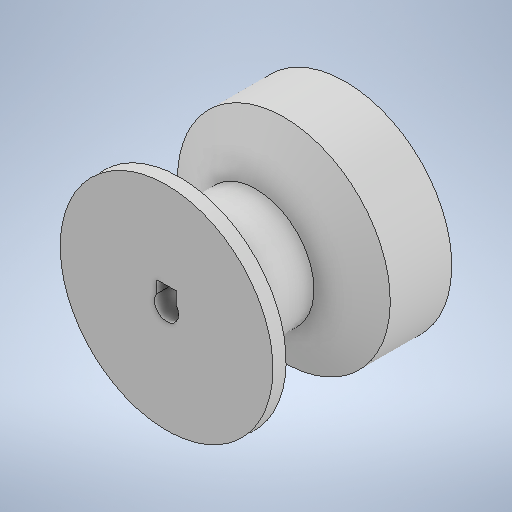
# Autodesk Inventor part: Vbelt Drive Pulley
Saved by Autodesk Inventor 2025 (Build 290162010, 162A)
## iProperties
Created: 2024-08-22
Part Number: Vbelt Drive Pulley
Material: Generic
Document SubType Name: Modeling
Designer: max_d
Density: 1 g/cm^3
Appearance: Default
Author: max_d
Autodesk Inventor part; units mm, degrees
ref_plane "YZ Plane" through (0, 0, 0) normal (1, 0, 0) x (0, 1, 0)
ref_plane "XZ Plane" through (0, 0, 0) normal (0, 1, 0) x (-1, 0, 0)
ref_plane "XY Plane" through (0, 0, 0) normal (0, 0, 1) x (1, 0, 0)
sketch "Sketch2" plane through (0, 0, 0) normal (1, 0, 0) x (0, 1, 0)
  line L0 (0, 0) -> (12, 0) construction
  line L1 (12, 0) -> (12, -5)
  line L2 (12, -5) -> (22, -10.7735)
  line L3 (22, -10.7735) -> (22, -13.5)
  line L4 (22, -13.5) -> (0, -13.5)
  line L5 (0, -13.5) -> (0, 0)
  line L6 (12, 0) -> (12, 5)
  line L7 (12, 5) -> (22, 10.7735)
  line L8 (22, 10.7735) -> (22, 13.5)
  line L9 (22, 13.5) -> (0, 13.5)
  line L10 (0, 13.5) -> (0, 0)
  line L11 (0, 0) -> (0, -46.5785) construction
  line L12 (22, -13.5) -> (22, -23.5)
  line L13 (22, -23.5) -> (0, -23.5)
  line L14 (0, -13.5) -> (0, -23.5)
  dimension "d0" = 22
  dimension "d1" = 13.5
  dimension "d2" = 5
  dimension "d3" = 60
  dimension "d4" = 10
  dimension "d16" = 10
  constraints: 30 end point, 4 symmetric about line, 3 perpendicular, 2 point on line, 2 vertical, 1 collinear, 1 horizontal, 1 parallel
  measures "d0" distance between parallel lines of L5 L3
  measures "d1" distance between parallel lines of L0 L4
  measures "d2" distance of L0.end L1.end
  measures "d3" angle of L1 L2
  measures "d4" distance between parallel lines of L3 L1
  measures "d16" distance of L3.end L12.end
revolve "Revolution1" add sketch "Sketch2" angle 360 about axis through (0, 0, 0) along (0, 0, -1)
sketch "Sketch3" plane through (0, 0, 13.5) normal (0, 0, 1) x (1, 0, 0)
  circle A0 centre (0, 0) radius 2.5
  line L0 (-2, 4) -> (2, 4)
  line L1 (2, 4) -> (2, -2.0439)
  line L2 (2, -2.0439) -> (-2, -2.0439)
  line L3 (-2, -2.0439) -> (-2, 4)
  line L4 (-2, 4) -> (2, -2.0439) construction
  line L5 (2, 4) -> (-2, -2.0439) construction
  line L6 (-5.2122, 2.5) -> (6.1572, 2.5) construction
  point P0 (0, 0.9781)
  point P1 (-2, 1.5)
  point P2 (2, 1.5)
  dimension "d6" = 5
  dimension "d7" = 4
  dimension "d9" = 1.5
  constraints: 14 end point, 2 horizontal, 2 midpoint, 2 parallel, 1 centre point, 1 coincident, 1 perpendicular, 1 tangent, 1 vertical alignment
  measures "d6" diameter of A0
  measures "d7" distance between parallel lines of L1 L3
  measures "d9" distance between parallel lines of L6 L0
extrude "Extrusion1" cut sketch "Sketch3" against normal through all contours A0 L1 | L1 A0 L2 L3 | A0 L3 L0 L1 | L3 A0 | A0 L2
sketch "Sketch4" plane through (0, 0, -23.5) normal (0, 0, 1) x (1, 0, 0)
  circle A0 centre (0, -17) radius 3
  arc A1 (-2, 1.5) -> (2, 1.5) centre (0, 0) ccw construction
  line L0 (0, 0) -> (0, -2.5) construction
  line L1 (0, -2.5) -> (0, -17) construction
  line L2 (0, -17) -> (0, -25) construction
  circle A2 centre (0, 0) radius 25 construction
  dimension "d12" = 6
  dimension "d17" = 8
  constraints: 6 end point, 2 vertical, 1 centre point, 1 point on circle, 1 point on line, 1 vertical alignment, 1 other
  measures "d12" diameter of A0
  measures "d17" distance of L1.end L2.end
body "Solid1"
